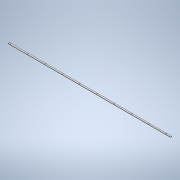
# Autodesk Inventor part: seguroAcrilico
Saved by Autodesk Inventor 2021.2 (Build 252289000, 289)
## iProperties
Created: 2026-07-28
Part Number: seguroAcrilico
Material: Generic
Document SubType Name: Sheet Metal
Designer: nelso
Density: 1 g/cm^3
Sheet Metal Rule: Default_mm
Appearance: Default
Author: nelso
Autodesk Inventor part; units mm, degrees
ref_plane "YZ Plane" through (0, 0, 0) normal (1, 0, 0) x (0, 1, 0)
ref_plane "XZ Plane" through (0, 0, 0) normal (0, 1, 0) x (-1, 0, 0)
ref_plane "XY Plane" through (0, 0, 0) normal (0, 0, 1) x (1, 0, 0)
sketch "Sketch1" plane through (0, 0, 0) normal (0, 1, 0) x (-1, 0, 0)
  line L0 (-750, 6.35) -> (750, 6.35)
  line L1 (750, 6.35) -> (750, -6.35)
  line L2 (750, -6.35) -> (-750, -6.35)
  line L3 (-750, -6.35) -> (-750, 6.35)
  line L4 (-750, 6.35) -> (750, -6.35) construction
  line L5 (750, 6.35) -> (-750, -6.35) construction
  line L6 (750, 0) -> (735, 0)
  circle A0 centre (735, 0) radius 3
  circle A1 centre (575, 0) radius 3
  circle A2 centre (415, 0) radius 3
  circle A3 centre (255, 0) radius 3
  circle A4 centre (95, 0) radius 3
  circle A5 centre (-65, 0) radius 3
  circle A6 centre (-225, 0) radius 3
  circle A7 centre (-385, 0) radius 3
  circle A8 centre (-545, 0) radius 3
  circle A9 centre (-705, 0) radius 3
  point P0 (0, 0)
  dimension "d0" = 1500
  dimension "d1" = 12.7
  dimension "d3" = 15
  dimension "d4" = 6
  dimension "d7" = 160
  measures "d0" distance of L1.end L2.end
  measures "d1" distance of L0.end L1.end
  measures "d3" distance of L6.start L6.end
  measures "d4" diameter of A0
  measures "d7" distance of A0.centre A1.centre
extrude "Plate1" add sketch "Sketch1" along normal blind 3.1 contours L0 L1 L2 L3 | A0 | A1 | A2 | A3 | A4 | A5 | A6 | A7 | A8 | A9
sketch "Sketch2" plane through (0, 3.1, 0) normal (0, 1, 0) x (1, 0, 0)
  line L0 (-750, -6.35) -> (-750, 6.35) projected
  line L1 (-750, 0) -> (-735, 0)
  circle A0 centre (-735, 0) radius 2.5
  circle A1 centre (-575, 0) radius 2.5
  circle A2 centre (-415, 0) radius 2.5
  circle A3 centre (-255, 0) radius 2.5
  circle A4 centre (-95, 0) radius 2.5
  circle A5 centre (65, 0) radius 2.5
  circle A6 centre (225, 0) radius 2.5
  circle A7 centre (385, 0) radius 2.5
  circle A8 centre (545, 0) radius 2.5
  circle A9 centre (705, 0) radius 2.5
  point P0 (0, 0)
  dimension "d12" = 15
  dimension "d13" = 5
  dimension "d16" = 160
  constraints: 10 centre point, 2 end point, 2 horizontal, 1 coincident, 1 midpoint, 18 other
  measures "d12" distance of L1.start L1.end
  measures "d13" diameter of A0
  measures "d16" distance of A0.centre A1.centre
extrude "Cut1" cut sketch "Sketch2" against normal blind 3.1
equation "\"d21\" = Thickness"
equation "\"d2\" = Thickness"
equation "\"BendRadius\" = Thickness"
equation "\"BendReliefWidth\" = Thickness"
equation "\"BendReliefDepth\" = 0.5 * Thickness"
equation "\"CornerReliefSize\" = 4 * Thickness"
equation "\"MinimumRemnant\" = 2 * Thickness"
equation "\"TransitionRadius\" = BendRadius"
equation "\"JacobiRadiusSize\" = BendRadius"
equation "\"GapSize\" = Thickness"
equation "\"Thickness\" = 3.1"
body "Solid1"
